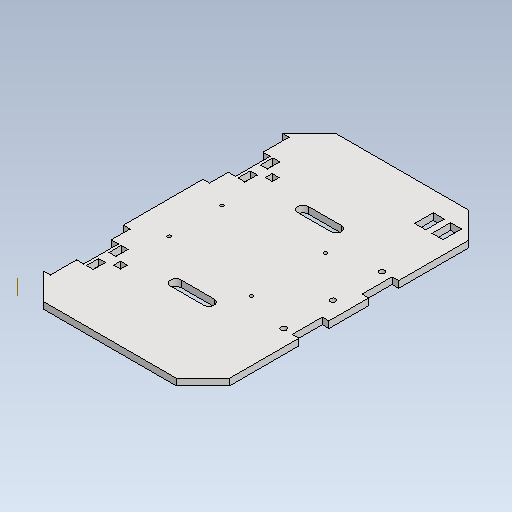
# Autodesk Inventor part: top-plate
Saved by Autodesk Inventor 2025 (Build 290162000, 162)
## iProperties
Created: 2025-08-20
Part Number: top-plate
Material: Generic
Document SubType Name: Modeling
Designer: HP
Density: 1 g/cm^3
Appearance: Default
Author: HP
Autodesk Inventor part; units mm, degrees
ref_plane "YZ Plane" through (0, 0, 0) normal (1, 0, 0) x (0, 1, 0)
ref_plane "XZ Plane" through (0, 0, 0) normal (0, 1, 0) x (-1, 0, 0)
ref_plane "XY Plane" through (0, 0, 0) normal (0, 0, 1) x (1, 0, 0)
sketch "Sketch1" plane through (0, 0, 0) normal (0, 1, 0) x (-1, 0, 0)
  line L0 (145, 110) -> (-145, 110)
  line L1 (-145, 110) -> (-145, -110)
  line L2 (-145, -110) -> (145, -110)
  line L3 (145, -110) -> (145, 110)
  line L4 (145, 110) -> (-145, -110) construction
  line L5 (-145, 110) -> (145, -110) construction
  line L6 (105, -80.8333) -> (35, -80.8333)
  line L7 (35, -80.8333) -> (35, -115.8333)
  line L8 (35, -115.8333) -> (105, -115.8333)
  line L9 (105, -115.8333) -> (105, -80.8333)
  line L10 (105, -80.8333) -> (35, -115.8333) construction
  line L11 (35, -80.8333) -> (105, -115.8333) construction
  line L12 (-35, -115.8333) -> (-105, -115.8333)
  line L13 (-105, -115.8333) -> (-105, -80.8333)
  line L14 (-105, -80.8333) -> (-35, -80.8333)
  line L15 (-35, -80.8333) -> (-35, -115.8333)
  line L16 (-35, -115.8333) -> (-105, -80.8333) construction
  line L17 (-105, -115.8333) -> (-35, -80.8333) construction
  line L18 (0, 110) -> (0, -110) construction
  line L19 (5, -110) -> (5, 110)
  point P0 (0, 0)
  point P1 (70, -98.3333)
  point P2 (-70, -98.3333)
  point P3 (0, 0)
  point P4 (-105, -110)
  point P5 (-35, -110)
  point P6 (-15, -80.8333)
  point P7 (-55, -80.8333)
  point P8 (105, -110)
  point P9 (35, -110)
  dimension "d1" = 70
  dimension "d2" = 70
  dimension "d3" = 35
  dimension "d4" = 35
  dimension "d5" = 140
  dimension "d6" = 11.6667
  dimension "d7" = 220
  dimension "d8" = 290
  dimension "d34" = 140
  constraints: 40 end point, 8 midpoint, 6 parallel, 3 horizontal, 3 perpendicular, 2 point on line, 1 coincident, 1 horizontal alignment, 1 vertical, 1 other
  measures "d1" distance between parallel lines of L7 L9
  measures "d2" distance between parallel lines of L13 L15
  measures "d3" distance between parallel lines of L6 L8
  measures "d4" distance between parallel lines of L14 L12
  measures "d5" distance of point (-70, -98.333) point (70, -98.333)
  measures "d6" distance from line of L2 point (70, -98.333)
  measures "d7" distance between parallel lines of L0 L2
  measures "d8" distance between parallel lines of L1 L3
  measures "d34" distance between parallel lines of L3 L19
extrude "Extrusion1" add sketch "Sketch1" along normal blind 5 contours L3 L2 L9 L6 L7 L19 L0 | L2 L7 L6 L9
sketch "Sketch5" plane through (0, 5, 0) normal (0, 1, 0) x (1, 0, 0)
  line L0 (-145, -110) -> (-5, -110) construction
  line L1 (-5, -110) -> (-5, 110) construction
  line L2 (-5, 110) -> (-145, 110) construction
  line L3 (-145, 110) -> (-145, -110) construction
  circle A0 centre (-120.5342, 20) radius 1.25
  circle A1 centre (-120.5342, -20) radius 1.25
  circle A2 centre (-50.5342, 28) radius 1.25
  circle A3 centre (-50.5342, -28) radius 1.25
  line L4 (-145, 0) -> (-5, 0) construction
  point P0 (0, 0)
  dimension "d35" = 56
  dimension "d36" = 40
  dimension "d37" = 70
  dimension "d38" = 2.5
  dimension "d39" = 2.5
  constraints: 4 centre point, 2 end point, 2 midpoint, 2 vertical alignment, 2 other
  measures "d35" distance of A3.centre A2.centre
  measures "d36" distance of A1.centre A0.centre
  measures "d37" horizontal distance of A2.centre A0.centre
  measures "d38" diameter of A0
  measures "d39" diameter of A2
extrude "Extrusion6" cut sketch "Sketch5" against normal through all
chamfer "Chamfer1" distance 20 angle 45 4 edges at (-145, 2.5, 110) (-145, 2.5, -110) (-5, 2.5, 110) (-5, 2.5, -110)
sketch "Sketch6" plane through (0, 5, 0) normal (0, 1, 0) x (1, 0, 0)
  circle A0 centre (-50.5342, -28) radius 1.25 projected
  circle A1 centre (-50.5342, 28) radius 1.25 projected
  circle A2 centre (-120.5342, -20) radius 1.25 projected
  circle A3 centre (-120.5342, 20) radius 1.25 projected
  line L0 (-25, 110) -> (-5, 90) projected
  line L1 (-25, 110) -> (-125, 110) projected
  line L2 (-145, 90) -> (-125, 110) projected
  line L3 (-145, 90) -> (-145, -90) projected
  line L4 (-125, -110) -> (-145, -90) projected
  line L5 (-125, -110) -> (-25, -110) projected
  line L6 (-5, -90) -> (-25, -110) projected
  line L7 (-5, -90) -> (-5, 90) projected
  line L8 (-145, 90) -> (-145, -90) projected
  line L9 (-5, 37.6) -> (-10, 37.6)
  line L10 (-10, 37.6) -> (-10, 15)
  line L11 (-10, 15) -> (-5, 15)
  line L12 (-5, 15) -> (-5, 37.6)
  line L13 (-5, 37.6) -> (-10, 15) construction
  line L14 (-10, 37.6) -> (-5, 15) construction
  line L15 (-5, -90) -> (-5, 90) projected
  line L16 (-87.5, 48) -> (-62.5, 48) construction
  line L17 (-87.5, 44) -> (-62.5, 44)
  line L18 (-62.5, 52) -> (-87.5, 52)
  arc A4 (-87.5, 52) -> (-87.5, 44) centre (-87.5, 48) ccw
  arc A5 (-62.5, 44) -> (-62.5, 52) centre (-62.5, 48) ccw
  line L19 (-145, 30) -> (-140, 30)
  line L20 (-140, 30) -> (-140, -30) construction
  line L21 (-140, -30) -> (-145, -30)
  line L22 (-145, -30) -> (-145, 30)
  line L23 (-145, 30) -> (-140, -30) construction
  line L24 (-140, 30) -> (-145, -30) construction
  line L25 (-140, 30) -> (-140, 95)
  line L26 (-140, -30) -> (-140, -95)
  line L27 (-145, 90) -> (-140, 90)
  point P0 (0, 0)
  point P1 (-7.5, 26.3)
  point P2 (-5, 15)
  point P3 (-5, 37.6)
  point P4 (-75, 48)
  point P5 (-75, 110)
  point P6 (-142.5, 0)
  point P7 (-145, 0)
  point P8 (-145, 0)
  dimension "d57" = 5
  dimension "d58" = 22.6
  dimension "d59" = 15
  dimension "d60" = 8
  dimension "d61" = 25
  dimension "d86" = 5
  dimension "d87" = 60
  dimension "d88" = 48
  constraints: 38 end point, 8 midpoint, 5 parallel, 4 point on circle, 4 tangent, 3 horizontal, 3 perpendicular, 3 point on line, 2 centre point, 2 collinear, 2 vertical, 1 horizontal alignment, 1 vertical alignment
  measures "d57" distance of L11.end L10.end
  measures "d58" distance of L10.end L9.end
  measures "d59" distance from line of point (0, 0) L11
  measures "d60" diameter of A5
  measures "d61" distance of L16.start L16.end
  measures "d86" distance between parallel lines of L20 L22
  measures "d87" distance between parallel lines of L21 L19
  measures "d88" distance from line of L16 point (-145, 0)
extrude "Extrusion7" cut sketch "Sketch6" against normal through all contours L7 L11 L10 L9 | L27 L25 L19 L3 | A4 L18 A5 L17
mirror "Mirror6" about plane through (0, 0, 0) normal (0, 0, 1) of "Extrusion7"
sketch "Sketch8" plane through (0, 5, 0) normal (0, 1, 0) x (1, 0, 0)
  circle A0 centre (-120.5342, 20) radius 1.25 construction
  circle A1 centre (-120.5342, -20) radius 1.25 construction
  circle A2 centre (-50.5342, 28) radius 1.25 construction
  circle A3 centre (-50.5342, -28) radius 1.25 construction
  line L0 (-87.5, 52) -> (-62.5, 52) construction
  arc A4 (-62.5, 44) -> (-62.5, 52) centre (-62.5, 48) ccw construction
  line L1 (-62.5, 44) -> (-87.5, 44) construction
  arc A5 (-87.5, 52) -> (-87.5, 44) centre (-87.5, 48) ccw construction
  line L2 (-87.5, -44) -> (-62.5, -44) construction
  arc A6 (-62.5, -52) -> (-62.5, -44) centre (-62.5, -48) ccw construction
  line L3 (-62.5, -52) -> (-87.5, -52) construction
  arc A7 (-87.5, -44) -> (-87.5, -52) centre (-87.5, -48) ccw construction
  line L4 (-125, -110) -> (-145, -90) construction
  line L5 (-125, -110) -> (-25, -110) construction
  line L6 (-5, -90) -> (-25, -110) construction
  line L7 (-5, -90) -> (-5, -37.6) construction
  line L8 (-5, -37.6) -> (-10, -37.6) construction
  line L9 (-10, -37.6) -> (-10, -15) construction
  line L10 (-10, -15) -> (-5, -15) construction
  line L11 (-5, -15) -> (-5, 15) construction
  line L12 (-5, 15) -> (-10, 15) construction
  line L13 (-10, 15) -> (-10, 37.6) construction
  line L14 (-10, 37.6) -> (-5, 37.6) construction
  line L15 (-5, 37.6) -> (-5, 90) construction
  line L16 (-25, 110) -> (-5, 90) construction
  line L17 (-25, 110) -> (-125, 110) construction
  line L18 (-145, 90) -> (-125, 110) construction
  line L19 (-145, 30) -> (-145, -30) construction
  line L20 (-23.3, 95) -> (-15, 95)
  line L21 (-15, 95) -> (-15, 81)
  line L22 (-15, 81) -> (-23.3, 81)
  line L23 (-23.3, 81) -> (-23.3, 95)
  line L24 (-23.3, 95) -> (-15, 81) construction
  line L25 (-15, 95) -> (-23.3, 81) construction
  line L26 (-36.3, 95) -> (-28, 95)
  line L27 (-28, 95) -> (-28, 81)
  line L28 (-28, 81) -> (-36.3, 81)
  line L29 (-36.3, 81) -> (-36.3, 95)
  line L30 (-36.3, 95) -> (-28, 81) construction
  line L31 (-28, 95) -> (-36.3, 81) construction
  line L32 (-132.6, -44.1) -> (-127.4, -44.1)
  line L33 (-127.4, -44.1) -> (-127.4, -53.3)
  line L34 (-127.4, -53.3) -> (-132.6, -53.3)
  line L35 (-132.6, -53.3) -> (-132.6, -44.1)
  line L36 (-132.6, -44.1) -> (-127.4, -53.3) construction
  line L37 (-127.4, -44.1) -> (-132.6, -53.3) construction
  line L38 (-132.6, -61.1) -> (-127.4, -61.1)
  line L39 (-127.4, -61.1) -> (-127.4, -70.3)
  line L40 (-127.4, -70.3) -> (-132.6, -70.3)
  line L41 (-132.6, -70.3) -> (-132.6, -61.1)
  line L42 (-132.6, -61.1) -> (-127.4, -70.3) construction
  line L43 (-127.4, -61.1) -> (-132.6, -70.3) construction
  line L44 (-117.4, -54.6) -> (-122.6, -54.6)
  line L45 (-122.6, -54.6) -> (-122.6, -59.8)
  line L46 (-122.6, -59.8) -> (-117.4, -59.8)
  line L47 (-117.4, -59.8) -> (-117.4, -54.6)
  line L48 (-117.4, -54.6) -> (-122.6, -59.8) construction
  line L49 (-122.6, -54.6) -> (-117.4, -59.8) construction
  line L50 (-130, -48.7) -> (-130, -65.7) construction
  line L51 (-140, -44.1) -> (-134.6, -44.1)
  line L52 (-134.6, -44.1) -> (-134.6, -70.3)
  line L53 (-134.6, -70.3) -> (-140, -70.3)
  line L54 (-140, -70.3) -> (-140, -44.1)
  line L55 (-140, -44.1) -> (-134.6, -70.3) construction
  line L56 (-134.6, -44.1) -> (-140, -70.3) construction
  line L57 (-140, 90) -> (-140, 30) projected
  line L58 (-140, 30) -> (-145, 30) projected
  line L59 (-145, -30) -> (-140, -30) projected
  line L60 (-140, -30) -> (-140, -90) projected
  circle A8 centre (-17.1, 0) radius 2.1
  circle A9 centre (-17.1, 37) radius 2.1
  circle A10 centre (-17.1, -37) radius 2.1
  point P0 (0, 0)
  point P1 (-19.15, 88)
  point P2 (-32.15, 88)
  point P3 (-120, -57.2)
  point P4 (-130, -57.2)
  point P5 (-137.3, -57.2)
  point P6 (-140, 95)
  point P7 (-140, -95)
  dimension "d63" = 14
  dimension "d64" = 8.3
  dimension "d65" = 14
  dimension "d66" = 8.3
  dimension "d67" = 13
  dimension "d68" = 15
  dimension "d69" = 10
  dimension "d72" = 52.8
  dimension "d73" = 10
  dimension "d74" = 9.2
  dimension "d75" = 9.2
  dimension "d76" = 5.2
  dimension "d77" = 5.2
  dimension "d78" = 5.2
  dimension "d79" = 5.2
  dimension "d80" = 15
  dimension "d81" = 17
  dimension "d83" = 2
  dimension "d89" = 4.2
  dimension "d90" = 4.2
  dimension "d91" = 4.2
  dimension "d92" = 17.1
  dimension "d93" = 37
  dimension "d94" = 37
  constraints: 74 end point, 13 midpoint, 12 parallel, 11 centre point, 6 horizontal, 6 perpendicular, 4 horizontal alignment, 3 vertical alignment, 2 collinear, 1 vertical
  measures "d63" distance between parallel lines of L22 L20
  measures "d64" distance between parallel lines of L23 L21
  measures "d65" distance between parallel lines of L28 L26
  measures "d66" distance between parallel lines of L29 L27
  measures "d67" distance of point (-32.15, 88) point (-19.15, 88)
  measures "d68" distance between parallel lines of L17 L20
  measures "d69" distance between parallel lines of L15 L21
  measures "d72" distance from line of L5 point (-120, -57.2)
  measures "d73" distance from line of point (-120, -57.2) L50
  measures "d74" distance between parallel lines of L34 L32
  measures "d75" distance between parallel lines of L40 L38
  measures "d76" distance between parallel lines of L35 L33
  measures "d77" distance between parallel lines of L41 L39
  measures "d78" distance between parallel lines of L45 L47
  measures "d79" distance between parallel lines of L46 L44
  measures "d80" distance between parallel lines of L19 L50
  measures "d81" distance of L50.end L50.start
  measures "d83" distance between parallel lines of L35 L52
  measures "d89" diameter of A8
  measures "d90" diameter of A9
  measures "d91" diameter of A10
  measures "d92" distance of point (0, 0) A8.centre
  measures "d93" distance of A8.centre A9.centre
  measures "d94" distance of A10.centre A8.centre
extrude "Extrusion8" cut sketch "Sketch8" against normal through all contours L20 L21 L22 L23 | L26 L27 L28 L29 | A8 | A9 | A10
extrude "Extrusion9" cut sketch "Sketch8" against normal through all contours L32 L33 L34 L35 | L38 L39 L40 L41 | L47 L46 L45 L44 | L51 L52 L53 L54
mirror "Mirror7" about plane through (0, 0, 0) normal (0, 0, 1) of "Extrusion9"
equation "\"d2\" = d1"
equation "\"d4\" = d3"
equation "\"d6\" = 0.333333 * d3"
equation "\"d39\" = d38"
equation "\"d65\" = d63"
equation "\"d66\" = d64"
equation "\"d75\" = d74"
equation "\"d77\" = d76"
equation "\"d90\" = d89"
equation "\"d91\" = d89"
equation "\"d94\" = d93"
body "Solid1"
